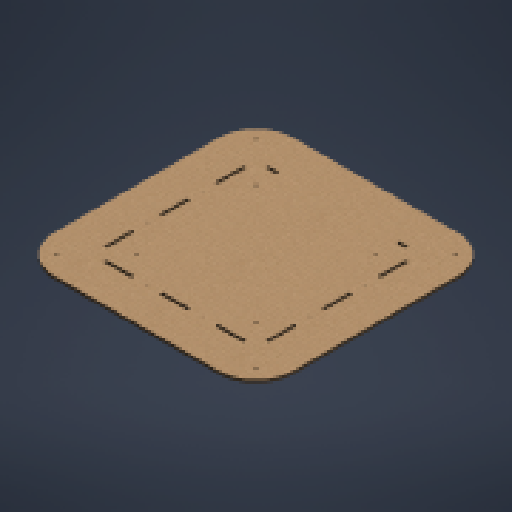
# Autodesk Inventor part: Baseplate
Saved by Autodesk Inventor 2024.1 (Build 281209000, 209)
## iProperties
Created: 2023-08-03
Part Number: Baseplate
Material: MDF Medium Density Fiberboard
Document SubType Name: Modeling
Designer: jaege
Density: 0.8 g/cm^3
Appearance: Cardboard - Corrugated
Mass: 276.45 g
Surface Area: 1816.12 cm^2
Volume: 345.562 cm^3
Author: jaege
Autodesk Inventor part; units mm, degrees
ref_plane "YZ Plane" through (0, 0, 0) normal (1, 0, 0) x (0, 1, 0)
ref_plane "XZ Plane" through (0, 0, 0) normal (0, 1, 0) x (-1, 0, 0)
ref_plane "XY Plane" through (0, 0, 0) normal (0, 0, 1) x (1, 0, 0)
sketch "Sketch1" plane through (0, 0, 0) normal (0, 1, 0) x (-1, 0, 0)
  line L0 (-104, 150) -> (104, 150)
  line L1 (150, 104) -> (150, -104)
  line L2 (104, -150) -> (-104, -150)
  line L3 (-150, -104) -> (-150, 104)
  line L4 (-150, 150) -> (150, -150) construction
  line L5 (150, 150) -> (-150, -150) construction
  line L6 (-100, 100) -> (100, 100) construction
  line L7 (100, 100) -> (100, -100) construction
  line L8 (100, -100) -> (-100, -100) construction
  line L9 (-100, -100) -> (-100, 100) construction
  line L10 (-100, 100) -> (100, -100) construction
  line L11 (100, 100) -> (-100, -100) construction
  line L12 (-125, 125) -> (125, 125) construction
  line L13 (125, 125) -> (125, -125) construction
  line L14 (125, -125) -> (-125, -125) construction
  line L15 (-125, -125) -> (-125, 125) construction
  line L16 (-125, 125) -> (125, -125) construction
  line L17 (125, 125) -> (-125, -125) construction
  line L18 (-75, 75) -> (75, 75) construction
  line L19 (75, 75) -> (75, -75) construction
  line L20 (75, -75) -> (-75, -75) construction
  line L21 (-75, -75) -> (-75, 75) construction
  line L22 (-75, 75) -> (75, -75) construction
  line L23 (75, 75) -> (-75, -75) construction
  line L24 (-104, -104) -> (104, -104) construction
  line L25 (104, -104) -> (104, 104) construction
  line L26 (104, 104) -> (-104, 104) construction
  line L27 (-104, 104) -> (-104, -104) construction
  circle A0 centre (125, -125) radius 1.5
  circle A1 centre (75, -75) radius 1.5
  circle A2 centre (75, 75) radius 1.5
  circle A3 centre (125, 125) radius 1.5
  circle A4 centre (-75, 75) radius 1.5
  circle A5 centre (-125, 125) radius 1.5
  circle A6 centre (-75, -75) radius 1.5
  circle A7 centre (-125, -125) radius 1.5
  line L28 (17.5, -100) -> (-17.5, -100)
  line L29 (-17.5, -100) -> (-17.5, -104)
  line L30 (-17.5, -104) -> (17.5, -104)
  line L31 (17.5, -104) -> (17.5, -100)
  arc A8 (104, -150) -> (150, -104) centre (104, -104) ccw
  arc A9 (150, 104) -> (104, 150) centre (104, 104) ccw
  arc A10 (-150, -104) -> (-104, -150) centre (-104, -104) ccw
  arc A11 (-104, 150) -> (-150, 104) centre (-104, 104) ccw
  line L32 (87.5, -100) -> (52.5, -100)
  line L33 (52.5, -100) -> (52.5, -104)
  line L34 (52.5, -104) -> (87.5, -104)
  line L35 (87.5, -104) -> (87.5, -100)
  line L36 (-87.5, -100) -> (-52.5, -100)
  line L37 (-52.5, -100) -> (-52.5, -104)
  line L38 (-52.5, -104) -> (-87.5, -104)
  line L39 (-87.5, -104) -> (-87.5, -100)
  line L40 (52.5, -104) -> (17.5, -100) construction
  line L41 (-17.5, -100) -> (-52.5, -104) construction
  line L42 (100, 17.5) -> (100, -17.5)
  line L43 (104, -17.5) -> (104, 17.5)
  line L44 (104, 17.5) -> (100, 17.5)
  line L45 (100, 52.5) -> (104, 52.5)
  line L46 (100, 87.5) -> (100, 52.5)
  line L47 (104, 87.5) -> (100, 87.5)
  line L48 (104, 52.5) -> (104, 87.5)
  line L49 (104, 52.5) -> (100, 17.5) construction
  line L50 (100, -17.5) -> (104, -17.5)
  line L51 (100, -17.5) -> (104, -52.5) construction
  line L52 (100, -52.5) -> (104, -52.5)
  line L53 (104, -87.5) -> (100, -87.5)
  line L54 (104, -52.5) -> (104, -87.5)
  line L55 (100, -87.5) -> (100, -52.5)
  line L56 (-17.5, 100) -> (17.5, 100)
  line L57 (17.5, 104) -> (-17.5, 104)
  line L58 (-17.5, 104) -> (-17.5, 100)
  line L59 (-52.5, 100) -> (-52.5, 104)
  line L60 (-87.5, 100) -> (-52.5, 100)
  line L61 (-87.5, 104) -> (-87.5, 100)
  line L62 (-52.5, 104) -> (-87.5, 104)
  line L63 (-52.5, 104) -> (-17.5, 100) construction
  line L64 (17.5, 100) -> (17.5, 104)
  line L65 (17.5, 100) -> (52.5, 104) construction
  line L66 (52.5, 100) -> (52.5, 104)
  line L67 (87.5, 104) -> (87.5, 100)
  line L68 (52.5, 104) -> (87.5, 104)
  line L69 (87.5, 100) -> (52.5, 100)
  line L70 (-100, -17.5) -> (-100, 17.5)
  line L71 (-104, 17.5) -> (-104, -17.5)
  line L72 (-104, -17.5) -> (-100, -17.5)
  line L73 (-100, -52.5) -> (-104, -52.5)
  line L74 (-100, -87.5) -> (-100, -52.5)
  line L75 (-104, -87.5) -> (-100, -87.5)
  line L76 (-104, -52.5) -> (-104, -87.5)
  line L77 (-104, -52.5) -> (-100, -17.5) construction
  line L78 (-100, 17.5) -> (-104, 17.5)
  line L79 (-100, 17.5) -> (-104, 52.5) construction
  line L80 (-100, 52.5) -> (-104, 52.5)
  line L81 (-104, 87.5) -> (-100, 87.5)
  line L82 (-104, 52.5) -> (-104, 87.5)
  line L83 (-100, 87.5) -> (-100, 52.5)
  point P0 (0, 0)
  point P1 (0, -100)
  point P2 (87.5, -102)
  point P3 (100, 0)
  point P4 (102, 87.5)
  point P5 (0, 100)
  point P6 (-87.5, 102)
  point P7 (-100, 0)
  point P8 (-102, -87.5)
  dimension "d0" = 300
  dimension "d1" = 300
  dimension "d2" = 200
  dimension "d3" = 200
  dimension "d4" = 4
  dimension "d5" = 25
  dimension "d6" = 25
  dimension "d7" = 3
  dimension "d8" = 3
  dimension "d11" = 360
  dimension "d16" = 4
  dimension "d24" = 46
  dimension "d25" = 46
  dimension "d31" = 35
  dimension "d32" = 35
  dimension "d35" = 360
  constraints: 168 end point, 16 parallel, 15 point on line, 12 centre point, 10 midpoint, 8 perpendicular, 8 point on circle, 8 tangent, 7 horizontal, 3 equal length, 2 coincident, 2 equal radius, 1 vertical alignment, 133 other
  measures "d0" distance of L4.end L5.end
  measures "d1" distance of L5.start L4.end
  measures "d2" distance of L7.end L8.end
  measures "d3" distance of L6.end L7.end
  measures "d4" distance between parallel lines of L8 L24
  measures "d5" distance between parallel lines of L1 L13
  measures "d6" distance between parallel lines of L7 L19
  measures "d7" diameter of A0
  measures "d8" diameter of A1
  measures "d16" distance of L29.end L28.end
  measures "d24" radius of A9
  measures "d25" radius of A8
  measures "d31" distance of L30.end L33.end
  measures "d32" distance of L29.end L30.end
extrude "Extrusion1" add sketch "Sketch1" along normal blind 4
sketch "Sketch3" plane through (0, 0, 0) normal (0, -1, 0) x (1, 0, 0)
  circle A0 centre (-35, 102) radius 1.5
  circle A1 centre (35, 102) radius 1.5
  line L0 (-52.5, 104) -> (-17.5, 100) construction
  line L1 (17.5, 100) -> (52.5, 104) construction
  circle A2 centre (-102, -35) radius 1.5
  circle A3 centre (-102, 35) radius 1.5
  circle A4 centre (35, -102) radius 1.5
  circle A5 centre (-35, -102) radius 1.5
  circle A6 centre (102, 35) radius 1.5
  circle A7 centre (102, -35) radius 1.5
  point P0 (0, 0)
  dimension "d44" = 3
  dimension "d45" = 3
  dimension "d48" = 360
  constraints: 8 centre point, 4 end point, 2 midpoint, 17 other
  measures "d44" diameter of A0
  measures "d45" diameter of A1
extrude "Extrusion2" cut sketch "Sketch3" against normal up to next
sketch "Sketch4" plane through (0, 0, 0) normal (0, -1, 0) x (1, 0, 0)
  line L0 (87.5, -100) -> (-87.5, -100)
  line L1 (-87.5, -100) -> (-87.5, -104)
  line L2 (-87.5, -104) -> (-75, -104)
  line L3 (-75, -104) -> (-75, -135)
  line L4 (-75, -135) -> (75, -135)
  line L5 (75, -135) -> (75, -104)
  line L6 (75, -104) -> (87.5, -104)
  line L7 (87.5, -104) -> (87.5, -100)
  circle A0 centre (102, 35) radius 1.5
  circle A1 centre (-102, -35) radius 1.5
  circle A2 centre (-35, 102) radius 1.5
  circle A3 centre (102, -35) radius 1.5
  circle A4 centre (-102, 35) radius 1.5
  circle A5 centre (35, 102) radius 1.5
  circle A6 centre (125, -125) radius 1.5
  circle A7 centre (125, 125) radius 1.5
  circle A8 centre (-125, 125) radius 1.5
  circle A9 centre (-125, -125) radius 1.5
  line L8 (100, 17.5) -> (100, -17.5)
  line L9 (100, -17.5) -> (104, -17.5)
  line L10 (104, -17.5) -> (104, 17.5)
  line L11 (104, 17.5) -> (100, 17.5)
  line L12 (100, 52.5) -> (104, 52.5)
  line L13 (104, 52.5) -> (104, 87.5)
  line L14 (104, 87.5) -> (100, 87.5)
  line L15 (100, 87.5) -> (100, 52.5)
  line L16 (100, -52.5) -> (100, -87.5)
  line L17 (100, -87.5) -> (104, -87.5)
  line L18 (104, -87.5) -> (104, -52.5)
  line L19 (104, -52.5) -> (100, -52.5)
  line L20 (-17.5, 100) -> (17.5, 100)
  line L21 (17.5, 100) -> (17.5, 104)
  line L22 (17.5, 104) -> (-17.5, 104)
  line L23 (-17.5, 104) -> (-17.5, 100)
  line L24 (-52.5, 100) -> (-52.5, 104)
  line L25 (-52.5, 104) -> (-87.5, 104)
  line L26 (-87.5, 104) -> (-87.5, 100)
  line L27 (-87.5, 100) -> (-52.5, 100)
  line L28 (52.5, 100) -> (87.5, 100)
  line L29 (87.5, 100) -> (87.5, 104)
  line L30 (87.5, 104) -> (52.5, 104)
  line L31 (52.5, 104) -> (52.5, 100)
  line L32 (-100, -17.5) -> (-100, 17.5)
  line L33 (-100, 17.5) -> (-104, 17.5)
  line L34 (-104, 17.5) -> (-104, -17.5)
  line L35 (-104, -17.5) -> (-100, -17.5)
  line L36 (-100, -52.5) -> (-104, -52.5)
  line L37 (-104, -52.5) -> (-104, -87.5)
  line L38 (-104, -87.5) -> (-100, -87.5)
  line L39 (-100, -87.5) -> (-100, -52.5)
  line L40 (-100, 52.5) -> (-100, 87.5)
  line L41 (-100, 87.5) -> (-104, 87.5)
  line L42 (-104, 87.5) -> (-104, 52.5)
  line L43 (-104, 52.5) -> (-100, 52.5)
  circle A10 centre (-75, -75) radius 1.5
  circle A11 centre (-75, 75) radius 1.5
  circle A12 centre (75, 75) radius 1.5
  circle A13 centre (75, -75) radius 1.5
  arc A14 (-150, -104) -> (-104, -150) centre (-104, -104) ccw
  line L44 (-150, -104) -> (-150, 104)
  arc A15 (-104, 150) -> (-150, 104) centre (-104, 104) ccw
  line L45 (-104, 150) -> (104, 150)
  arc A16 (150, 104) -> (104, 150) centre (104, 104) ccw
  line L46 (150, 104) -> (150, -104)
  arc A17 (104, -150) -> (150, -104) centre (104, -104) ccw
  line L47 (104, -150) -> (-104, -150)
  circle A18 centre (-102, 35) radius 1.5 projected
  circle A19 centre (102, -35) radius 1.5 projected
  circle A20 centre (35, -102) radius 1.5 projected
  circle A21 centre (35, 102) radius 1.5 projected
  circle A22 centre (-102, -35) radius 1.5 projected
  circle A23 centre (102, 35) radius 1.5 projected
  circle A24 centre (-35, -102) radius 1.5 projected
  circle A25 centre (-35, 102) radius 1.5 projected
  circle A26 centre (-125, -125) radius 1.5 projected
  circle A27 centre (-125, 125) radius 1.5 projected
  circle A28 centre (125, 125) radius 1.5 projected
  circle A29 centre (125, -125) radius 1.5 projected
  line L48 (17.5, -100) -> (-17.5, -100) projected
  line L49 (-17.5, -100) -> (-17.5, -104) projected
  line L50 (-17.5, -104) -> (17.5, -104) projected
  line L51 (17.5, -104) -> (17.5, -100) projected
  line L52 (-52.5, -100) -> (-87.5, -100) projected
  line L53 (-87.5, -100) -> (-87.5, -104) projected
  line L54 (-87.5, -104) -> (-52.5, -104) projected
  line L55 (-52.5, -104) -> (-52.5, -100) projected
  line L56 (87.5, -104) -> (87.5, -100) projected
  line L57 (87.5, -100) -> (52.5, -100) projected
  line L58 (52.5, -100) -> (52.5, -104) projected
  line L59 (52.5, -104) -> (87.5, -104) projected
  line L60 (-100, -17.5) -> (-100, 17.5) projected
  line L61 (-100, 17.5) -> (-104, 17.5) projected
  line L62 (-104, 17.5) -> (-104, -17.5) projected
  line L63 (-104, -17.5) -> (-100, -17.5) projected
  line L64 (-104, 52.5) -> (-100, 52.5) projected
  line L65 (-100, 52.5) -> (-100, 87.5) projected
  line L66 (-100, 87.5) -> (-104, 87.5) projected
  line L67 (-104, 87.5) -> (-104, 52.5) projected
  line L68 (-100, -87.5) -> (-100, -52.5) projected
  line L69 (-100, -52.5) -> (-104, -52.5) projected
  line L70 (-104, -52.5) -> (-104, -87.5) projected
  line L71 (-104, -87.5) -> (-100, -87.5) projected
  line L72 (-17.5, 100) -> (17.5, 100) projected
  line L73 (17.5, 100) -> (17.5, 104) projected
  line L74 (17.5, 104) -> (-17.5, 104) projected
  line L75 (-17.5, 104) -> (-17.5, 100) projected
  line L76 (52.5, 104) -> (52.5, 100) projected
  line L77 (52.5, 100) -> (87.5, 100) projected
  line L78 (87.5, 100) -> (87.5, 104) projected
  line L79 (87.5, 104) -> (52.5, 104) projected
  line L80 (-87.5, 100) -> (-52.5, 100) projected
  line L81 (-52.5, 100) -> (-52.5, 104) projected
  line L82 (-52.5, 104) -> (-87.5, 104) projected
  line L83 (-87.5, 104) -> (-87.5, 100) projected
  line L84 (100, 17.5) -> (100, -17.5) projected
  line L85 (100, -17.5) -> (104, -17.5) projected
  line L86 (104, -17.5) -> (104, 17.5) projected
  line L87 (104, 17.5) -> (100, 17.5) projected
  line L88 (104, -52.5) -> (100, -52.5) projected
  line L89 (100, -52.5) -> (100, -87.5) projected
  line L90 (100, -87.5) -> (104, -87.5) projected
  line L91 (104, -87.5) -> (104, -52.5) projected
  line L92 (100, 87.5) -> (100, 52.5) projected
  line L93 (100, 52.5) -> (104, 52.5) projected
  line L94 (104, 52.5) -> (104, 87.5) projected
  line L95 (104, 87.5) -> (100, 87.5) projected
  circle A30 centre (75, -75) radius 1.5 projected
  circle A31 centre (75, 75) radius 1.5 projected
  circle A32 centre (-75, 75) radius 1.5 projected
  circle A33 centre (-75, -75) radius 1.5 projected
  arc A34 (104, -150) -> (150, -104) centre (104, -104) ccw projected
  line L96 (104, -150) -> (-104, -150) projected
  arc A35 (-150, -104) -> (-104, -150) centre (-104, -104) ccw projected
  line L97 (-150, -104) -> (-150, 104) projected
  arc A36 (-104, 150) -> (-150, 104) centre (-104, 104) ccw projected
  line L98 (-104, 150) -> (104, 150) projected
  arc A37 (150, 104) -> (104, 150) centre (104, 104) ccw projected
  line L99 (150, 104) -> (150, -104) projected
  line L100 (-75, -104) -> (-75, -100)
  line L101 (75, -104) -> (75, -100)
  point P0 (0, 0)
  constraints: 100 end point, 24 horizontal, 24 vertical, 18 centre point, 8 point on circle, 2 perpendicular, 2 point on line, 88 other
extrude "Extrusion3" add sketch "Sketch4" against normal up to surface (4 mm away) contours L101 L59 L58 L0 | L51 L50 L49 L0 | L55 L54 L100 L0 | A20 | A24
body "Solid1"
